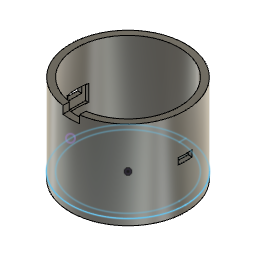
_top of base mic.5012af67-7226-4017-b96e-733cb6f4032c (Autodesk Fusion 360 design; units mm, degrees)
Autodesk Fusion 360 part; units mm, degrees
note: some values were not read from the file. Set by a fixed rule: which sketch regions a step uses.
sketch "Sketch1" plane through (0, 0, 0) normal (0, 0, 1) x (1, 0, 0)
  line L0 (21.25, 21.25) -> (-21.25, 21.25)
  line L1 (-21.25, 21.25) -> (-21.25, -21.25)
  line L2 (-21.25, -21.25) -> (21.25, -21.25)
  line L3 (21.25, -21.25) -> (21.25, 21.25)
  line L4 (21.25, 21.25) -> (-21.25, -21.25) construction
  line L5 (-21.25, 21.25) -> (21.25, -21.25) construction
  line L6 (25.25, -25.25) -> (-25.25, -25.25)
  line L7 (-25.25, -25.25) -> (-25.25, 25.25)
  line L8 (-25.25, 25.25) -> (25.25, 25.25)
  line L9 (25.25, 25.25) -> (25.25, -25.25)
  line L10 (25.25, -25.25) -> (-25.25, 25.25) construction
  line L11 (-25.25, -25.25) -> (25.25, 25.25) construction
  line L12 (-21.25, 0) -> (-25.25, 0)
  dimension "d2" = 42.5
  dimension "d3" = 42.5
  dimension "d4" = 4
  constraint horizontal L0
  constraint perpendicular L0 L1
  constraint parallel L0 L2
  constraint parallel L1 L3
  constraint coincident L4 origin
  constraint coincident L5 origin
  constraint horizontal L6
  constraint perpendicular L6 L7
  constraint parallel L6 L8
  constraint parallel L7 L9
  constraint coincident L10 origin
  constraint coincident L11 origin
  constraint midpoint L1 L12.start
  constraint midpoint L7 L12.end
  measures "d2" distance of L0.start L0.end
  measures "d3" distance of L0.end L1.end
  measures "d4" distance of L12.start L12.end
extrude "Extrude1" add sketch "Sketch1" along normal blind 3.2
sketch "Sketch2" plane through (0, 0, 0) normal (0, 0, 1) x (1, 0, 0)
  circle A0 centre (0, 0) radius 40.4366
  circle A1 centre (0, 0) radius 45.4366
  line L0 (0.1635, 40.4363) -> (0.1635, 45.4363)
  dimension "d7" = 5
  constraint coincident A0.centre A1.centre
  constraint coincident A0 L0.start
  constraint coincident A1 L0.end
  constraint vertical L0
  measures "d7" distance of L0.start L0.end
extrude "Extrude2" add sketch "Sketch2" against normal blind 5 contours A0 | A1
sketch "Sketch3" plane through (0, 0, 0) normal (0, 0, 1) x (1, 0, 0)
sketch "Sketch4" plane through (0, 0, 0) normal (0, 0, 1) x (1, 0, 0)
  line L0 (25.25, 25.25) -> (25.25, -25.25)
  line L1 (25.25, -25.25) -> (-25.25, -25.25)
  line L2 (-25.25, -25.25) -> (-25.25, 25.25)
  line L3 (-25.25, 25.25) -> (25.25, 25.25)
  circle A0 centre (0, 0) radius 45.4366
  circle A1 centre (0, 33.5) radius 5.5
extrude "Extrude3" cut sketch "Sketch4" against normal blind 10 contours A1
sketch "Sketch5" plane through (0, 0, 0) normal (0, 0, 1) x (1, 0, 0)
extrude "Extrude4" add sketch "Sketch2" along normal blind 64.5
sketch "Sketch6" plane through (0, 0, 0) normal (0, 0, 1) x (1, 0, 0)
  point P0 (-45.4366, 0)
ref_plane "WorkPlane1" through (0, 0, 64.5) normal (0, 0, 1) x (1, 0, 0)
sketch "Sketch7" plane through (0, 0, 64.5) normal (0, 0, 1) x (1, 0, 0)
  line L0 (-6.3568, -39.7886) -> (6.6432, -39.7886)
  line L1 (6.6432, -39.7886) -> (6.6432, -45.6886)
  line L2 (6.6432, -45.6886) -> (-6.3568, -45.6886)
  line L3 (-6.3568, -45.6886) -> (-6.3568, -39.7886)
  dimension "d15" = 5.9
  dimension "d16" = 13
  constraint horizontal L0
  constraint vertical L1
  constraint horizontal L2
  constraint vertical L3
  measures "d15" distance of L0.start L2.end
  measures "d16" distance of L0.start L0.end
extrude "Extrude5" cut sketch "Sketch7" against normal blind 6
sketch "Sketch8" plane through (0, 0, 0) normal (1, 0, 0) x (0, 1, 0)
  line L0 (-45.4366, 58.5) -> (-45.4366, -5)
  line L1 (45.4366, -5) -> (45.4366, 64.5)
  line L2 (0, 64.5) -> (0, -5) construction
  line L3 (-5.5, 34.75) -> (5.5, 34.75)
  line L4 (5.5, 34.75) -> (5.5, 29.75)
  line L5 (5.5, 29.75) -> (-5.5, 29.75)
  line L6 (-5.5, 29.75) -> (-5.5, 34.75)
  line L7 (45.4366, 64.5) -> (-44.9897, 64.5)
  line L8 (-45.4366, -5) -> (45.4366, -5)
  dimension "d19" = 11
  dimension "d20" = 5
  constraint vertical L2
  constraint horizontal L3
  constraint vertical L4
  constraint horizontal L5
  constraint vertical L6
  constraint coincident L2.start L7
  constraint coincident L2.end L8
  constraint midpoint L2 L5
  measures "d19" distance of L3.start L3.end
  measures "d20" distance of L3.start L5.end
extrude "Extrude6" cut sketch "Sketch8" along normal mid plane 200
sketch "Sketch9" plane through (0, 0, 0) normal (1, 0, 0) x (0, 1, 0)
  line L0 (-8.5, 36.25) -> (8.5, 36.25)
  line L1 (8.5, 36.25) -> (8.5, 23.25)
  line L2 (8.5, 23.25) -> (-8.5, 23.25)
  line L3 (-8.5, 23.25) -> (-8.5, 36.25)
  line L4 (0, 64.5) -> (0, -5)
  line L5 (-45.4366, -5) -> (45.4366, -5)
  line L6 (45.4366, 64.5) -> (-44.9897, 64.5)
  line L7 (0, 36.25) -> (0, 23.25)
  dimension "d23" = 17
  dimension "d24" = 13
  constraint horizontal L0
  constraint vertical L1
  constraint horizontal L2
  constraint vertical L3
  constraint vertical L4
  constraint coincident L4.end L5
  constraint coincident L4.start L6
  constraint midpoint L0 L7.start
  constraint midpoint L2 L7.end
  constraint midpoint L4 L7
  measures "d23" distance of L0.start L0.end
  measures "d24" distance of L0.end L1.end
extrude "Extrude7" cut sketch "Sketch9" along normal mid plane 84
